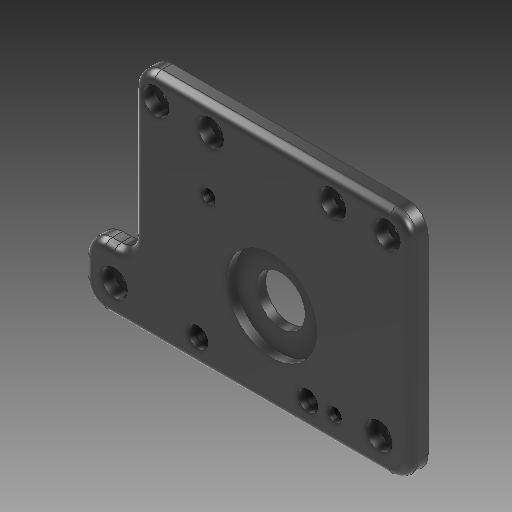
# Autodesk Inventor part: Extruder Motor Plate 2
Saved by Autodesk Inventor 2020.2 (Build 242310000, 310)
## iProperties
Created: 2020-03-20
Part Number: Extruder Motor Plate 2
Material: ABS Plastic
Document SubType Name: Modeling
Designer: rah75
Density: 1.06 g/cm^3
Appearance: Satin - Black
Author: rah75
Title: Extruder Motor Plate
Autodesk Inventor part; units mm, degrees
ref_plane "YZ Plane" through (0, 0, 0) normal (1, 0, 0) x (0, 1, 0)
ref_plane "XZ Plane" through (0, 0, 0) normal (0, 1, 0) x (-1, 0, 0)
ref_plane "XY Plane" through (0, 0, 0) normal (0, 0, 1) x (1, 0, 0)
sketch "Sketch1" plane through (0, 0, 0) normal (0, 0, 1) x (1, 0, 0)
  line L0 (-40, -28.4) -> (40, -28.4)
  line L1 (40, -28.4) -> (40, 28.4)
  line L2 (40, 28.4) -> (-40, 28.4)
  line L3 (-40, 28.4) -> (-40, -28.4)
  line L4 (-40, -28.4) -> (40, 28.4) construction
  line L5 (40, -28.4) -> (-40, 28.4) construction
  line L6 (-32.5, -20.9) -> (32.5, -20.9) construction
  line L7 (32.5, -20.9) -> (32.5, 20.9) construction
  line L8 (32.5, 20.9) -> (-32.5, 20.9) construction
  line L9 (-32.5, 20.9) -> (-32.5, -20.9) construction
  line L10 (-32.5, -20.9) -> (32.5, 20.9) construction
  line L11 (32.5, -20.9) -> (-32.5, 20.9) construction
  circle A0 centre (-32.5, -20.9) radius 3.25 construction
  circle A1 centre (32.5, 20.9) radius 3.25 construction
  circle A2 centre (32.5, -20.9) radius 3.25 construction
  line L12 (-40, -13.4) -> (-27.8, -13.4)
  line L13 (-27.8, -13.4) -> (-27.8, 28.4)
  circle A3 centre (-20.3, 20.9) radius 3.25 construction
  line L14 (40, 28.4) -> (32.5, 20.9)
  line L15 (-27.8, 28.4) -> (-20.3, 20.9) construction
  point P0 (0, 0)
  point P1 (34.5, 22.9)
  point P2 (-22.3, 22.9)
  dimension "d0" = 80
  dimension "d1" = 56.8
  dimension "d2" = 41.8
  dimension "d3" = 65
  dimension "d4" = 6.5
  dimension "d5" = 6.5
  dimension "d6" = 6.5
  dimension "d8" = 7.5
  dimension "d9" = 7.5
  dimension "d10" = 7.5
  dimension "d11" = 12.2
  dimension "d12" = 6.5
  dimension "d13" = 7.5
  dimension "d61" = 5.5
  dimension "d62" = 5.5
  constraints: 32 end point, 5 point on line, 4 centre point, 4 midpoint, 4 parallel, 3 coincident, 3 horizontal, 3 perpendicular
  measures "d0" distance of L2.end L1.end
  measures "d1" distance of L1.end L0.end
  measures "d2" distance of L7.end L6.end
  measures "d3" distance of L7.end L8.end
  measures "d4" diameter of A0
  measures "d5" diameter of A1
  measures "d6" diameter of A2
  measures "d8" distance between parallel lines of L3 L9
  measures "d9" distance between parallel lines of L8 L2
  measures "d10" distance from line of L6.start L12
  measures "d11" distance between parallel lines of L3 L13
  measures "d12" diameter of A3
  measures "d13" distance from line of L13 L15.end
  measures "d61" distance from line of point (34.5, 22.9) L1
  measures "d62" distance from line of L13 point (-22.3, 22.9)
extrude "Base" add sketch "Sketch1" against normal blind 4.5 contours L3 L12 L13 L2 L1 L0
hole "Main Holes" at (32.5, -20.9, 0) at (-32.5, -20.9, 0) at (34.5, 22.9, 0) at (-22.3, 22.9, 0) direction (0, 0, -1) diameter 3.4 end through all counterbore diameter 6.5 counterbore depth 3 clearance for "Socket Head Cap Screw" size "M3" standard "Ansi Metric M Profile"
fillet "Fillet1" radius 5 6 edges at (-40, -28.4, -2.25) (-40, -13.4, -2.25) (-27.8, -13.4, -2.25) (-27.8, 28.4, -2.25) (40, 28.4, -2.25) (40, -28.4, -2.25)
sketch "Sketch2" plane through (0, 0, 0) normal (0, 0, 1) x (1, 0, 0)
  circle A0 centre (32.5, -20.9) radius 1.7 projected
  point P0 (0, 0)
  point P1 (6.1, -6.4)
  point P2 (6.1, 11.6)
  dimension "d24" = 6.1
  dimension "d25" = 14.5
  dimension "d26" = 18
  constraints: 1 vertical alignment
  measures "d24" horizontal distance of point (6.1, -6.4) point (0, 0)
  measures "d25" vertical distance of A0.centre point (6.1, -6.4)
  measures "d26" distance of point (6.1, -6.4) point (6.1, 11.6)
hole "Motor Bore" at (6.1, -6.4, 0) direction (0, 0, -1) diameter 12 end through all counterbore diameter 22.25 counterbore depth 2.25
sketch "Sketch3" plane through (0, 0, -4.5) normal (0, 0, -1) x (-1, 0, 0)
  circle A0 centre (-6.1, -6.4) radius 6 projected
  point P0 (0, 0)
  point P1 (-6.1, 11.6)
  dimension "d34" = 18
  constraints: 1 vertical alignment
  measures "d34" distance of A0.centre point (-6.1, 11.6)
hole "Hole3" at (6.1, 11.6, -4.5) direction (0, 0, 1) diameter 13 depth 2.5 counterbore diameter 16.25 counterbore depth 2
sketch "Sketch4" plane through (-35, -28.4, 0) normal (0, -1, 0) x (1, 0, 0)
  circle A0 centre (35, -12.25) radius 8.5
  line L0 (0, 0) -> (70, 0) projected
  line L1 (70, -4.5) -> (0, -4.5) projected
  point P0 (35, 0)
  point P1 (35, 0)
  dimension "d43" = 17
  dimension "d50" = 7.75
  constraints: 1 centre point, 1 midpoint, 1 vertical alignment
  measures "d43" diameter of A0
  measures "d50" distance from line of L1 A0.centre
extrude "Extrusion2" cut sketch "Sketch4" against normal blind 10
sketch "Sketch5" plane through (-35, -28.4, -4.5) normal (0, -1, 0) x (1, 0, 0)
  line L0 (4.5, 2.75) -> (65.5, 2.75)
  line L1 (65.5, 2.75) -> (65.5, 0)
  line L2 (65.5, 0) -> (4.5, 0)
  line L3 (4.5, 0) -> (4.5, 2.75)
  line L4 (4.5, 2.75) -> (65.5, 0) construction
  line L5 (65.5, 2.75) -> (4.5, 0) construction
  line L6 (70, 0) -> (0, 0) projected
  point P0 (35, 4.5)
  point P1 (35, 1.375)
  point P2 (35, 0)
  dimension "d46" = 61
  dimension "d47" = 2.75
  constraints: 12 end point, 4 midpoint, 2 parallel, 1 horizontal, 1 perpendicular
  measures "d46" distance of L1.end L2.end
  measures "d47" distance of L0.end L1.end
extrude "Extrusion3" cut sketch "Sketch5" against normal blind 2.5
fillet "Fillet2" radius 2 9 edges at (-26.3355, 26.9355, 0) (-27.8, 7.5, 0) (-29.2645, -11.9355, 0) (-38.5355, -26.9355, 0) (0, -28.4, 0) (38.5355, -26.9355, 0) (40, 0, 0) (38.5355, 26.9355, 0) (6.1, 28.4, 0)
sketch "Sketch6" plane through (0, 0, -4.5) normal (0, 0, -1) x (-1, 0, 0)
  circle A0 centre (-6.1, -6.4) radius 6 projected
  line L0 (-21.6, 9.1) -> (9.4, 9.1) construction
  line L1 (9.4, 9.1) -> (9.4, -21.9) construction
  line L2 (9.4, -21.9) -> (-21.6, -21.9) construction
  line L3 (-21.6, -21.9) -> (-21.6, 9.1) construction
  line L4 (-21.6, 9.1) -> (9.4, -21.9) construction
  line L5 (9.4, 9.1) -> (-21.6, -21.9) construction
  point P0 (0, 0)
  dimension "d52" = 31
  constraints: 12 end point, 4 coincident, 2 midpoint, 2 parallel, 2 perpendicular, 1 horizontal
  measures "d52" distance of L0.end L1.end
hole "Hole4" at (-9.4, 9.1, -4.5) at (21.6, -21.9, -4.5) direction (0, 0, 1) diameter 3.4 end through all counterbore diameter 6.5 counterbore depth 3 clearance for "Socket Head Cap Screw" size "M3" standard "Ansi Metric M Profile"
sketch "Sketch8" plane through (0, 0, 0) normal (0, 0, 1) x (1, 0, 0)
  circle A0 centre (-9.4, 9.1) radius 1.7 projected
  circle A1 centre (34.5, 22.9) radius 3.25 projected
  circle A2 centre (32.5, -20.9) radius 3.25 projected
  circle A3 centre (-32.5, -20.9) radius 3.25 projected
  circle A4 centre (-22.3, 22.9) radius 3.25 projected
  circle A5 centre (6.1, -6.4) radius 11.125 projected
  arc A6 (-22.8, 26.4) -> (-25.8, 23.4) centre (-22.8, 23.4) ccw projected
  line L0 (-25.8, -8.4) -> (-25.8, 23.4) projected
  arc A7 (-32.8, -15.4) -> (-25.8, -8.4) centre (-32.8, -8.4) ccw projected
  line L1 (-35, -15.4) -> (-32.8, -15.4) projected
  arc A8 (-35, -15.4) -> (-38, -18.4) centre (-35, -18.4) ccw projected
  line L2 (-38, -23.4) -> (-38, -18.4) projected
  arc A9 (-38, -23.4) -> (-35, -26.4) centre (-35, -23.4) ccw projected
  line L3 (35, -26.4) -> (-35, -26.4) projected
  arc A10 (35, -26.4) -> (38, -23.4) centre (35, -23.4) ccw projected
  line L4 (38, 23.4) -> (38, -23.4) projected
  arc A11 (38, 23.4) -> (35, 26.4) centre (35, 23.4) ccw projected
  line L5 (-22.8, 26.4) -> (35, 26.4) projected
  line L6 (-8.9, 22.9) -> (21.1, 22.9)
  point P0 (0, 0)
  point P1 (6.1, 22.9)
  dimension "d63" = 30
  constraints: 2 coincident, 2 end point, 1 horizontal, 1 midpoint, 1 point on line, 1 vertical alignment
  measures "d63" distance of L6.start L6.end
hole "Hole5" at (-8.9, 22.9, 0) at (21.1, 22.9, 0) direction (0, 0, -1) diameter 3.4 end through all counterbore diameter 6.5 counterbore depth 3 clearance for "Socket Head Cap Screw" size "M3" standard "Ansi Metric M Profile"
sketch "Sketch9" plane through (0, 0, -4.5) normal (0, 0, -1) x (-1, 0, 0)
  line L0 (30.5, -28.3843) -> (-30.5, -28.3843) projected
  point P0 (0, 0)
  point P1 (-15, -22.1843)
  point P2 (12, -22.1843)
  dimension "d71" = 15
  dimension "d72" = 12
  dimension "d73" = 6.2
  constraints: 1 horizontal alignment
  measures "d71" horizontal distance of point (-15, -22.184) point (0, 0)
  measures "d72" horizontal distance of point (12, -22.184) point (0, 0)
  measures "d73" distance from line of point (-15, -22.184) L0
hole "Hole6" at (15, -22.1843, -4.5) at (-12, -22.1843, -4.5) direction (0, 0, 1) diameter 5 end through all countersink diameter 5.4 countersink angle 8
equation "\"d13\" = d10"
body "Solid1"
